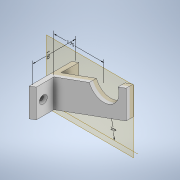
# Autodesk Inventor part: PipeSupport-2_00-020
Saved by Autodesk Inventor 2021.1 (Build 251245000, 245)
## iProperties
Created: 2020-09-15
Part Number: PipeSupport-2_00-020
Material: Generic
Document SubType Name: Modeling
Designer: robst
Density: 1 g/cm^3
Appearance: Default
Author: robst
Autodesk Inventor part; units mm, degrees
ref_plane "YZ Plane" through (0, 0, 0) normal (1, 0, 0) x (0, 1, 0)
ref_plane "XZ Plane" through (0, 0, 0) normal (0, 1, 0) x (-1, 0, 0)
sketch "Sketch5" plane through (0, 0, 0) normal (0, 0, 1) x (1, 0, 0)
  line L0 (0, 0) -> (6.35, 0)
  line L1 (6.35, 0) -> (6.35, 25.4)
  line L2 (6.35, 25.4) -> (0, 25.4)
  line L3 (0, 25.4) -> (0, 0)
  dimension "d21" = 25.4
  dimension "d22" = 6.35
  constraints: 8 end point, 2 parallel, 1 horizontal, 1 perpendicular
  measures "d21" distance from line of L2 L0.start
  measures "d22" distance from line of L1 L0.start
extrude "Extrusion3" add sketch "Sketch5" against normal mid plane 38.1
sketch "Sketch6" plane through (0, 0, 0) normal (0, 0, 1) x (1, 0, 0)
  line L0 (6.35, 25.4) -> (6.35, 0) projected
  line L1 (0, 25.4) -> (6.35, 25.4) projected
  line L2 (6.35, 0) -> (0, 0) projected
  line L3 (0, 0) -> (0, 25.4) projected
  line L4 (6.35, 0) -> (70.8025, 23.4588)
  line L5 (6.35, 0) -> (74.9389, 0) construction
  line L6 (70.8025, 48.8588) -> (70.8025, 23.4588)
  arc A0 (37.9708, 36.909) -> (63.6292, 46.2479) centre (50.8, 41.5785) ccw
  line L7 (6.35, 25.4) -> (37.9708, 36.909)
  line L8 (63.6292, 46.2479) -> (70.8025, 48.8588)
  dimension "d25" = 20
  dimension "d26" = 27.305
  dimension "d29" = 6.35
  dimension "d30" = 50.8
  dimension "d33" = 0
  constraints: 10 end point, 2 parallel, 2 point on circle, 1 centre point, 1 collinear, 1 equal length, 1 horizontal, 1 vertical
  measures "d25" angle of L5 L4
  measures "d26" diameter of A0
  measures "d29" distance edge to line of A0 L6
  measures "d30" distance from line of A0.centre L3
  measures "d33" distance from line of L7 A0.centre
extrude "Extrusion4" add sketch "Sketch6" along normal mid plane 6.35 contours L7 A0 L8 L6 L4 L0
sketch "Sketch7" plane through (6.35, 0, 19.05) normal (1, 0, 0) x (0, 0, -1)
  line L0 (38.1, 25.4) -> (0, 25.4) construction
  line L1 (6.35, 25.4) -> (6.35, 0) construction
  line L2 (31.75, 25.4) -> (31.75, 0) construction
  line L3 (0, 0) -> (0, 25.4) construction
  line L4 (38.1, 25.4) -> (38.1, 0) construction
  line L5 (0, 0) -> (15.875, 0) projected
  line L6 (22.225, 0) -> (38.1, 0) projected
  point P0 (19.05, 0)
  point P1 (6.35, 12.7)
  point P2 (31.75, 12.7)
  dimension "d34" = 6.35
  dimension "d35" = 6.35
  constraints: 4 end point, 2 midpoint, 2 point on line, 2 vertical
  measures "d34" distance between parallel lines of L1 L3
  measures "d35" distance between parallel lines of L2 L4
sketch "Sketch8" plane through (0, 0, 0) normal (0, 0, 1) x (1, 0, 0)
  line L0 (0, 0) -> (0, 25.4) projected
  line L1 (6.35, 0) -> (0, 0) projected
  line L2 (70.8025, 23.4588) -> (6.35, 0) projected
  line L3 (0, 0) -> (6.35, 0)
  line L4 (0, -2.3112) -> (6.35, 0)
  line L5 (0, 0) -> (0, -2.3112)
  constraints: 6 end point, 2 collinear, 1 vertical
extrude "Extrusion5" add sketch "Sketch8" along normal mid plane 38.1
hole "Hole3" at (6.35, 12.7, 12.7) at (6.35, 12.7, -12.7) direction (-1, 0, 0) diameter 3.81 end through all countersink diameter 7.0866 countersink angle 82 clearance for "Flat Head Machine Screw (82)" size "#6" standard "Ansi Unified Screw Threads"
sketch "Sketch9" plane through (0, 0, 0) normal (0, 0, 1) x (1, 0, 0)
  line L0 (0, -2.3112) -> (0, 25.4) projected
  line L1 (0, 25.4) -> (6.35, 25.4) projected
  line L2 (6.35, 25.4) -> (37.9708, 36.909) projected
  line L3 (6.35, 25.4) -> (6.35, 0) projected
  line L4 (6.35, 25.4) -> (0, 25.4)
  line L5 (6.35, 25.4) -> (6.35, 0) projected
  line L6 (6.35, 25.4) -> (0, 23.0888)
  line L7 (0, 25.4) -> (0, 23.0888)
  point P0 (0, 0)
  constraints: 6 end point, 3 collinear, 1 point on line
extrude "Extrusion6" cut sketch "Sketch9" along normal mid plane 38.1
equation "\"d21\" = supportHeight"
equation "\"d22\" = supportWidth"
equation "\"d23\" = totalScrewHoldWidth"
equation "\"d25\" = supportAngle"
equation "\"d26\" = pipeDiameter"
equation "\"d30\" = distanceFromWallToPipeCenter"
equation "\"d31\" = supportWidth"
equation "\"d47\" = totalScrewHoldWidth"
equation "\"d62\" = totalScrewHoldWidth"
equation "\"pipeDiameter\" = 27.305"
equation "\"distanceFromWallToPipeCenter\" = 50.8"
equation "\"supportHeight\" = 25.4"
equation "\"supportWidth\" = 6.35"
equation "\"screwHoldDepth\" = 6.35"
equation "\"totalScrewHoldWidth\" = 38.1"
equation "\"screwPositionFromTop\" = 6.35"
equation "\"supportAngle\" = 20deg"
body "Solid1"
body "Solid2"
